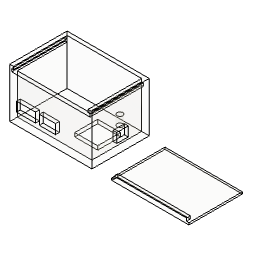
ESP01 Relay (Autodesk Fusion 360 design; units mm, degrees)
Autodesk Fusion 360 part; units mm, degrees
note: some values were not read from the file. Chosen so that the rebuilt part matches the saved one: which face or edge a step refers to; which pieces of a blend or face edit are solid.
sketch "Sketch1" plane through (0, 0, 0) normal (0, 0, 1) x (1, 0, 0)
box "BoxPrimitive2" add length 30 width 43 height 24 placed x (0, 1, 0) y (-1, 0, 0) z (0, 0, 1) at (43, 0, 0) makes body 1
shell "Shell1" thickness 2 removed faces 1 at (14.3333, 10, 24) on bodies 1
cylinder "CylinderPrimitive1" add diameter 3 height 5 placed x (1, 0, 0) y (0, 1, 0) z (0, 0, 1) at (7.4578, 25.9289, 2) bodies 1
move_face "MoveFace1" to x (1, 0, 0) y (0, 1, 0) z (0, 0, 1) at (28, 0, 0) 2 faces at (8.9503, 25.7796, 5.3333) (7.8738, 26.0521, 7) on bodies 1
move_face "MoveFace2" to x (1, 0, 0) y (0, 1, 0) z (0, 0, 1) at (-2.96, 0, 0) 1 faces at (35.9355, 27.3508, 5.3333) on bodies 1
move_face "MoveFace3" to x (1, 0, 0) y (0, 1, 0) z (0, 0, 1) at (0, -0.55, 0) 1 faces at (33.3734, 24.711, 3.6667) on bodies 1
box "BoxPrimitive3" add length 5 width 20 height 5 placed x (0, 0, -1) y (1, 0, 0) z (0, -1, 0) at (57.9696, 0, 15.6772) separate body makes body 2
move_body "Move1" bodies 2 to x (1, 0, 0) y (0, 1, 0) z (0, 0, 1) at (-54, 0, -5)
move_face "MoveFace4" by (0, 0, -1.68) 5 faces at (10.6363, -1.6667, 10.6772) (10.6363, -1.6667, 5.6772) (3.9696, -1.6667, 7.3438) (23.9696, -1.6667, 7.3438) (17.3029, 0, 9.0105) on bodies 2
move_face "MoveFace5" by (-0.47, 0, 0) 1 faces at (3.9696, -3.3333, 7.3305) on bodies 2
move_face "MoveFace6" by (0, 3, 0) 3 faces at (3.4996, -3.3333, 7.3305) (10.3229, -5, 7.3305) (23.9696, -3.3333, 7.3305) on bodies 2
extrude "Extrude1" cut 1 faces at (10.3229, -2, 7.3305) along direction (0, 1, 0) blind 5 on bodies 2 bodies 1 2
box "BoxPrimitive4" cut length 4 width 6 height -2 placed x (0, 0, -1) y (0, 1, 0) z (1, 0, 0) at (43, 14, 7) bodies 1
move_face "MoveFace7" by (0, -5, 0) 1 faces at (41.6667, 20, 4.3333) on bodies 1
move_face "MoveFace8" by (0, -5, 0) 1 faces at (41.6667, 14, 4.3333) on bodies 1
move_face "MoveFace9" by (0, -2, 0) 1 faces at (41.6667, 9, 4.3333) on bodies 1
move_face "MoveFace10" by (0, -2, 0) 1 faces at (41.6667, 15, 4.3333) on bodies 1
move_face "MoveFace11" by (0, 0, 1) 1 faces at (41.6667, 9, 3) on bodies 1
move_face "MoveFace12" by (0, 0, 1) 1 faces at (41.6667, 9, 7) on bodies 1
box "BoxPrimitive5" cut length 11 width 11 height -2 placed x (0, 1, 0) y (1, 0, 0) z (0, 0, -1) at (27, 8, 0) bodies 1
move_face "MoveFace13" by (0, 6, 0) 1 faces at (41.6667, 13, 5.3333) on bodies 1
move_face "MoveFace14" by (0, 6, 0) 2 faces at (41.6667, 11, 8) (41.6667, 7, 5.3333) on bodies 1
move_face "MoveFace15" by (0, 0, 1) 1 faces at (10.3229, 0.6667, 3.9972) on bodies 1
move_face "MoveFace16" by (0, 0, 1) 1 faces at (17.1463, 0.6667, 8.9972) on bodies 1
move_face "MoveFace17" by (0, 0, 1) 1 faces at (41.6667, 15, 8) on bodies 1
move_face "MoveFace18" by (-3, 0, 0) 1 faces at (27, 15.3333, 1.3333) on bodies 1
move_face "MoveFace19" by (0, 3, 0) 1 faces at (28.6667, 19, 1.3333) on bodies 1
move_face "MoveFace20" by (-2, 0, 0) 1 faces at (38, 17.3333, 1.3333) on bodies 1
move_face "MoveFace21" by (0, 2, 0) 1 faces at (28, 8, 1.3333) on bodies 1
move_face "MoveFace22" to x (1, 0, 0) y (0, 1, 0) z (0, 0, 1) at (0, -0.5, 0) 1 faces at (32.9755, 26.8008, 5.3333) on bodies 1
move_face "MoveFace23" to x (1, 0, 0) y (0, 1, 0) z (0, 0, 1) at (0, 0.25, 0) 1 faces at (32.9755, 26.3008, 5.3333) on bodies 1
box "BoxPrimitive6" cut length 2 width 39 height -2 placed x (0, 0, 1) y (-1, 0, 0) z (0, -1, 0) at (41, 0, 22) bodies 1
box "BoxPrimitive7" cut length 1 width 28 height -1 placed x (0, 0, 1) y (0, -1, 0) z (1, 0, 0) at (2, 28, 22) bodies 1
box "BoxPrimitive8" cut length 1 width 28 height -1 placed x (0, 0, -1) y (0, -1, 0) z (-1, 0, 0) at (41, 28, 23) bodies 1
box "BoxPrimitive9" add length 28 width 41 height 1 placed x (0, 1, 0) y (-1, 0, 0) z (0, 0, 1) at (94, 0, 0) separate body makes body 3
box "BoxPrimitive10" add length 2 width 39 height 1 placed x (0, 1, 0) y (-1, 0, 0) z (0, 0, 1) at (93, 0, 1) bodies 2 3
move_face "MoveFace24" by (-0.5, 0, 0) 1 faces at (93, 1.3333, 1.3333) on bodies 2
move_face "MoveFace25" by (0.5, 0, 0) 1 faces at (54, 1.3333, 1.3333) on bodies 2
move_face "MoveFace26" by (0.25, 0, 0) 1 faces at (53, 18.6667, 0.3333) on bodies 2
move_face "MoveFace27" by (-0.25, 0, 0) 1 faces at (94, 18.6667, 0.3333) on bodies 2
move_face "MoveFace28" by (0, 0, -0.5) 1 faces at (15, 0.6667, 22) on bodies 1
move_face "MoveFace29" by (0, 0, 0.5) 1 faces at (67.1667, 0.6667, 2) on bodies 2
move_face "MoveFace30" by (0, 0, 1) 1 faces at (10.3229, 0.6667, 4.9972) on bodies 1
move_face "MoveFace31" by (0, 0, 1) 1 faces at (42.3333, 17, 4) on bodies 1
move_face "MoveFace32" by (0, 0, 1) 1 faces at (41.6667, 15, 9) on bodies 1
move_face "MoveFace33" by (0, 0, 1) 1 faces at (17.1463, 0.6667, 9.9972) on bodies 1
box "BoxPrimitive11" add length 5 width 2 height -2 placed x (0, 0, 1) y (-1, 0, 0) z (0, -1, 0) at (15.0235, 0, 5.9972) bodies 1
move_face "MoveFace34" by (0.48, 0, 0) 1 faces at (15.0235, 1.3333, 9.3305) on bodies 1
move_face "MoveFace35" by (0.48, 0, 0) 1 faces at (13.0235, 1.3333, 9.3305) on bodies 1
move_face "MoveFace36" by (0, 0, 2) 1 faces at (15, 29.3333, 24) on bodies 1
move_face "MoveFace37" by (0, 0, 1.5) 3 faces at (1.3333, 10, 23) (2, 0.6667, 24.3333) (2, 19.3333, 24.3333) on bodies 1
move_face "MoveFace38" by (0, 0, 1.5) 3 faces at (41.6667, 10, 23) (41, 0.6667, 24.3333) (41, 19.3333, 24.3333) on bodies 1
move_face "MoveFace39" by (0, 0, 1.5) 2 faces at (1, 18.6667, 22.5) (15, 0.6667, 21.5) on bodies 1
